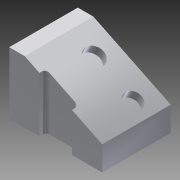
# Autodesk Inventor part: 8.2 Q2
Saved by Autodesk Inventor 2015 (Build 190159000, 159)
## iProperties
Created: 2018-04-11
Part Number: 8.2 Q2
Material: Aluminum 6061
Document SubType Name: Modeling
Designer: Administrator
Density: 2.7 g/cm^3
Appearance: Aluminum - Flat
Mass: 209.857 g
Surface Area: 392.15 cm^2
Volume: 77.7247 cm^3
Author: Administrator
Autodesk Inventor part; units mm, degrees
ref_plane "YZ Plane" through (0, 0, 0) normal (1, 0, 0) x (0, 1, 0)
ref_plane "XZ Plane" through (0, 0, 0) normal (0, 1, 0) x (-1, 0, 0)
ref_plane "XY Plane" through (0, 0, 0) normal (0, 0, 1) x (1, 0, 0)
sketch "Sketch1" plane through (0, 0, 0) normal (0, 0, 1) x (1, 0, 0)
  line L0 (0, 0) -> (0, 59.2667)
  line L1 (0, 59.2667) -> (14.8167, 59.2667)
  line L2 (14.8167, 59.2667) -> (88.9, 23.2833)
  line L3 (88.9, 23.2833) -> (88.9, 0)
  line L4 (88.9, 0) -> (0, 0)
  dimension "OverallHeight" = 59.2667
  dimension "TopWidth" = 14.8167
  dimension "RightHeight" = 23.2833
  dimension "OverallWidth" = 88.9
  constraints: 10 end point, 1 parallel, 1 perpendicular
  measures "OverallHeight" distance of L0.start L0.end
  measures "TopWidth" distance of L0.end L1.end
  measures "RightHeight" distance of L2.end L3.end
  measures "OverallWidth" distance of L3.end L0.start
extrude "Extrusion1" add sketch "Sketch1" along normal blind 65.6167
sketch "Sketch2" plane through (14.8167, 59.2667, 65.6167) normal (0.436904, 0.8995082, 0) x (0.8995082, -0.436904, 0)
  circle A0 centre (25.2098, 43.7444) radius 8.9958
  circle A1 centre (66.4848, 43.7444) radius 8.2021
  line L0 (0, 65.6167) -> (82.3598, 65.6167) projected
  line L1 (82.3598, 65.6167) -> (82.3598, 0) projected
  point P0 (12.5661, 65.6167)
  dimension "UpperHoleDiameter" = 17.9917
  dimension "LowerHoleDiameter" = 16.4042
  dimension "EdgeDistance" = 15.875
  dimension "HoleAllignment" = 0
  dimension "HoleToCenter" = 41.275
  dimension "BackEdgeToHoleCenters" = 21.8722
  constraints: 2 centre point
  measures "UpperHoleDiameter" diameter of A0
  measures "LowerHoleDiameter" diameter of A1
  measures "EdgeDistance" distance from line of L1 A1.centre
  measures "HoleAllignment" vertical distance of A1.centre A0.centre
  measures "HoleToCenter" distance of A1.centre A0.centre
  measures "BackEdgeToHoleCenters" distance from line of L0 A1.centre
extrude "Extrusion2" cut sketch "Sketch2" against normal blind 8.2021
sketch "Sketch3" plane through (14.8167, 59.2667, 65.6167) normal (0.436904, 0.8995082, 0) x (0.8995082, -0.436904, 0)
  line L0 (82.3598, 0) -> (0, 0) projected
  line L1 (22.3523, 0) -> (53.4673, 0)
  line L2 (26.0565, 6.35) -> (49.7632, 6.35)
  line L3 (22.3523, 0) -> (22.3523, 2.6458)
  line L4 (53.4673, 2.6458) -> (53.4673, 0)
  line L5 (82.3598, 65.6167) -> (82.3598, 0) projected
  arc A0 (26.0565, 6.35) -> (22.3523, 2.6458) centre (26.0565, 2.6458) ccw
  arc A1 (53.4673, 2.6458) -> (49.7632, 6.35) centre (49.7632, 2.6458) ccw
  point P0 (12.5661, 65.6167)
  dimension "NotchWidth" = 31.115
  dimension "NotchDepth" = 6.35
  dimension "NotchLocation" = 28.8925
  dimension "d18" = 3.7042
  constraints: 8 end point, 4 point on circle, 4 tangent, 2 centre point, 2 point on line, 1 equal radius, 1 horizontal, 1 parallel, 1 vertical
  measures "NotchWidth" distance of L1.end L1.start
  measures "NotchDepth" distance between parallel lines of L0 L2
  measures "NotchLocation" distance between parallel lines of L4 L5
  measures "d18" radius of A0
sketch "Sketch4" plane through (0, 59.2667, 0) normal (0, 1, 0) x (1, 0, 0)
  line L0 (88.9, -65.6167) -> (0, -65.6167)
  line L1 (28.8925, -65.6167) -> (60.0075, -65.6167)
  line L2 (32.5967, -59.2667) -> (56.3033, -59.2667)
  line L3 (28.8925, -65.6167) -> (28.8925, -62.9708)
  line L4 (60.0075, -62.9708) -> (60.0075, -65.6167)
  line L5 (88.9, 57.15) -> (88.9, -65.6167)
  arc A0 (32.5967, -59.2667) -> (28.8925, -62.9708) centre (32.5967, -62.9708) ccw
  arc A1 (60.0075, -62.9708) -> (56.3033, -59.2667) centre (56.3033, -62.9708) ccw
  line L6 (14.8167, -65.6167) -> (0, -65.6167) projected
  line L7 (88.9, 0) -> (88.9, -65.6167) projected
  point P0 (0, 0)
  point P1 (11.3592, 57.15)
  dimension "d19" = 31.115
  dimension "d20" = 6.35
  dimension "d21" = 28.8925
  dimension "d22" = 3.7042
  dimension "d26" = 0
  dimension "d27" = 0
  constraints: 12 end point, 4 point on circle, 4 tangent, 2 centre point, 2 point on line, 1 equal radius, 1 horizontal, 1 parallel, 1 vertical
  measures "d19" distance of L1.end L1.start
  measures "d20" distance between parallel lines of L0 L2
  measures "d21" distance between parallel lines of L4 L5
  measures "d22" radius of A0
  measures "d26" distance between parallel lines of L6 L0
  measures "d27" distance between parallel lines of L7 L5
extrude "Extrusion3" cut sketch "Sketch4" against normal through all
shell "Shell1" thickness 4.101 removed faces 1 at (40.4989, 0, 19.7556)
equation "\"OverallWidth\" = 1.5 * OverallHeight"
equation "\"BackEdgeToHoleCenters\" = 0.333333 * Depth"
equation "\"HoleDepth\" = 0.5 * LowerHoleDiameter"
equation "\"NotchWidth\" = 0.35 * OverallWidth"
equation "\"NotchLocation\" = 0.5 * OverallWidth - 0.5 * NotchWidth"
equation "\"d18\" = 0.25 * TopWidth"
equation "\"d19\" = 0.35 * OverallWidth"
equation "\"d21\" = 0.5 * OverallWidth - 0.5 * d19"
equation "\"d22\" = 0.25 * TopWidth"
equation "\"d28\" = 0.5 * LowerHoleDiameter"
equation "\"ShellThickness\" = 0.5 * HoleDepth"
equation "\"d23\" = 1.5 * OverallHeight"
equation "\"d24\" = TopWidth"
equation "\"d25\" = OverallHeight"
equation "\"Depth\" = 65.616667"
body "Solid1"
